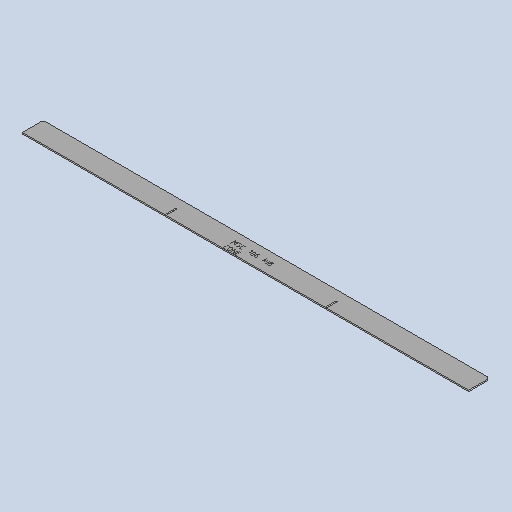
# Autodesk Inventor part: MSC 106 RIB CONE
Saved by Autodesk Inventor 2025 (Build 290162010, 162A)
## iProperties
Created: 2024-06-26
Part Number: MSC 106 RIB CONE
Material: Stainless Steel
Document SubType Name: Sheet Metal
Designer: pokla
Density: 8 g/cm^3
Sheet Metal Rule: AISI304 3mm Die 32
Appearance: Default
Stock Number: МОО 106 шпангоут конус
Mass: 1274.47 g
Surface Area: 1131.93 cm^2
Volume: 159.308 cm^3
Flat Pattern Width: 5 cm
Flat Pattern Length: 106.6 cm
Flat Pattern Area: 533 cm^2
Sheet Metal Width: 50,000 mm
Sheet Metal Length: 1066,000 mm
Sheet Metal Area: 53300,000 mm^2
Author: pokla
Autodesk Inventor part; units mm, degrees
ref_plane "YZ Plane" through (0, 0, 0) normal (1, 0, 0) x (0, 1, 0)
ref_plane "XZ Plane" through (0, 0, 0) normal (0, 1, 0) x (-1, 0, 0)
ref_plane "XY Plane" through (0, 0, 0) normal (0, 0, 1) x (1, 0, 0)
sketch "Sketch1" plane through (0, 0, 0) normal (0, 0, 1) x (1, 0, 0)
  line L0 (-600, 0) -> (600, 0)
  line L1 (-600, 0) -> (-600, 50)
  line L2 (-600, 50) -> (600, 50)
  line L3 (600, 50) -> (600, 0)
  circle A0 centre (-600, 0) radius 25
  circle A1 centre (600, 0) radius 25
  line L4 (600, 0) -> (644.2345, 16.1001)
  line L5 (644.2345, 16.1001) -> (635, 50)
  line L6 (635, 50) -> (600, 50)
  point P0 (0, 0)
  point P1 (0, 0)
  point P2 (-600, 25)
  point P3 (-575, 0)
  point P4 (575, 0)
  point P5 (600, 25)
  point P6 (623.4923, 8.5505)
  dimension "d18" = 50
  dimension "d19" = 1200
  dimension "d25" = 50
  dimension "d26" = 50
  dimension "d39" = 70
  dimension "d40" = 35
  measures "d18" distance of L2.end L0.end
  measures "d19" distance of L0.start L0.end
  measures "d25" diameter of A0
  measures "d26" diameter of A1
  measures "d39" angle of L3 L4
  measures "d40" distance of L2.end L5.end
extrude "Plate2" add sketch "Sketch1" against normal blind 3 contours L1 A0 L0 | A0 L1 L2 L3 A1 L0 | A1 L3 L0 picked at (-598.1457, 16.4577)
sketch "Sketch3" plane through (0, 0, 0) normal (0, 0, 1) x (1, 0, 0)
  line L0 (-191.55, 0) -> (-191.55, 50) construction
  line L1 (600, 50) -> (-600, 50) construction
  line L2 (-600, 50) -> (-600, 0) projected
  line L3 (-193.1, 26) -> (-190, 26)
  line L4 (-190, 26) -> (-190, 0)
  line L5 (-190, 0) -> (-193.1, 0)
  line L6 (-193.1, 0) -> (-193.1, 26)
  line L7 (-600, 0) -> (600, 0) projected
  line L8 (191.55, 50) -> (191.55, 0) construction
  line L9 (190, 26) -> (193.1, 26)
  line L10 (193.1, 26) -> (193.1, 0)
  line L11 (193.1, 0) -> (190, 0)
  line L12 (190, 0) -> (190, 26)
  line L13 (0, 0) -> (0, 50) construction
  point P0 (0, 0)
  point P1 (190, 0)
  point P2 (193.1, 0)
  dimension "d28" = 3.1
  dimension "d29" = 26
  dimension "d52" = 380
  constraints: 22 end point, 6 parallel, 5 midpoint, 4 point on line, 3 perpendicular, 2 horizontal, 1 vertical, 1 other
  measures "d28" distance of L4.end L5.end
  measures "d29" distance of L3.end L4.end
  measures "d52" distance between parallel lines of L12 L4
extrude "Extrusion2" cut sketch "Sketch3" against normal through all
sketch "Sketch4" plane through (0, 0, -3) normal (0, 0, -1) x (-1, 0, 0)
  line L0 (190, 0) -> (190, 26) projected
  line L1 (190, 26) -> (193.1, 26) projected
  line L2 (193.1, 26) -> (193.1, 0) projected
  line L3 (600, 0) -> (193.1, 0) projected
  line L4 (600, 50) -> (600, 0) projected
  line L5 (-600, 50) -> (600, 50) projected
  line L6 (-600, 0) -> (-600, 50) projected
  line L7 (-193.1, 0) -> (-600, 0) projected
  line L8 (-193.1, 0) -> (-193.1, 26) projected
  line L9 (-193.1, 26) -> (-190, 26) projected
  line L10 (-190, 26) -> (-190, 0) projected
  line L11 (190, 0) -> (-190, 0) projected
  line L12 (-533, 0) -> (-533, 50)
  line L13 (-600, 50) -> (600, 50) projected
  line L14 (600, 0) -> (193.1, 0) projected
  line L15 (533, 0) -> (533, 50)
  point P0 (0, 0)
  point P1 (533, 0)
  dimension "d45" = 67
  dimension "d46" = 67
  constraints: 4 end point, 4 point on line, 2 perpendicular
  measures "d45" distance between parallel lines of L4 L15
  measures "d46" distance between parallel lines of L6 L12
extrude "Extrusion3" cut sketch "Sketch4" against normal through all contours L15 L5 L4 L3 | L7 L6 L5 L12
sketch "Sketch5" plane through (0, 0, 0) normal (0, 0, 1) x (1, 0, 0)
  line L0 (-55.7541, 0.5014) -> (-55.7541, 31.0924) construction
  line L1 (-55.7541, 31.0924) -> (66.2742, 31.0924) construction
  line L2 (66.2742, 31.0924) -> (66.2742, 0.5014) construction
  line L3 (66.2742, 0.5014) -> (-55.7541, 0.5014) construction
  line L4 (533, 50) -> (-533, 50) projected
  line L5 (-533, 50) -> (-533, 0) projected
  point P0 (0, 0)
  constraints: 2 parallel, 2 other
mark "Mark1"
chamfer "Corner Chamfer1" distance 6 angle 45 2 edges at (-533, 50, -1.5) (533, 50, -1.5)
equation "\"d46\" = d45"
equation "\"d20\" = Thickness"
equation "\"BendReliefWidth\" = Thickness"
equation "\"BendReliefDepth\" = 0.5 * Thickness"
equation "\"CornerReliefSize\" = 4 * Thickness"
equation "\"MinimumRemnant\" = 2 * Thickness"
equation "\"TransitionRadius\" = BendRadius"
equation "\"JacobiRadiusSize\" = BendRadius"
equation "\"GapSize\" = Thickness"
equation "\"Thickness\" = 3"
equation "\"BendRadius\" = 5"
body "Solid2"
